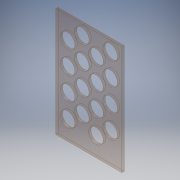
# Autodesk Inventor part: EBF_003.1-front-plate_cup-holder
Saved by Autodesk Inventor 2019 (Build 230136000, 136)
## iProperties
Created: 2019-02-28
Part Number: EBF_003.1-front-plate_cup-holder
Material: Generic
Document SubType Name: Modeling
Designer: Rene
Density: 1 g/cm^3
Appearance: Polycarbonate - Smoked
Author: Rene
Autodesk Inventor part; units mm, degrees
ref_plane "YZ Plane" through (0, 0, 0) normal (1, 0, 0) x (0, 1, 0)
ref_plane "XZ Plane" through (0, 0, 0) normal (0, 1, 0) x (-1, 0, 0)
ref_plane "XY Plane" through (0, 0, 0) normal (0, 0, 1) x (1, 0, 0)
sketch "Sketch1" plane through (0, 0, 0) normal (0, 0, 1) x (1, 0, 0)
  line L0 (-70, -115) -> (70, -115)
  line L1 (70, -115) -> (70, 115)
  line L2 (70, 115) -> (-70, 115)
  line L3 (-70, 115) -> (-70, -115)
  point P0 (0, 0)
  dimension "width" = 140
  dimension "d1" = 70
  dimension "d2" = 230
  dimension "d3" = 115
  constraints: 8 end point, 2 parallel, 1 horizontal, 1 perpendicular
  measures "width" distance of L0.start L0.end
  measures "d1" horizontal distance of point (0, 0) L0.start
  measures "d2" distance of L2.end L0.start
  measures "d3" vertical distance of point (0, 0) L0.start
extrude "Extrusion1" add sketch "Sketch1" along normal blind 5
sketch "Sketch2" plane through (0, 0, 5) normal (0, 0, 1) x (1, 0, 0)
  circle A0 centre (-45, 69) radius 15.5
  circle A1 centre (-15, 93) radius 15.5
  point P0 (0, 0)
  dimension "d6" = 31
  dimension "d7" = 69
  dimension "d8" = 45
  dimension "d17" = 31
  dimension "d18" = 30
  dimension "d19" = 24
  constraints: 2 centre point
  measures "d6" diameter of A0
  measures "d7" vertical distance of A0.centre point (0, 0)
  measures "d8" horizontal distance of A0.centre point (0, 0)
  measures "d17" diameter of A1
  measures "d18" horizontal distance of A1.centre A0.centre
  measures "d19" vertical distance of A1.centre A0.centre
extrude "Extrusion2" cut sketch "Sketch2" against normal blind 5
pattern_linear "Rectangular Pattern2" count 2 spacing 60 along (1, 0, 0) count 4 spacing 48 along (0, -1, 0) of "Extrusion2"
equation "\"d1\" = 0.5 * width"
equation "\"d3\" = 0.5 * d2"
equation "\"d17\" = d6"
equation "\"d22\" = 2 * d18"
equation "\"d25\" = 2 * d19"
body "Solid1"
